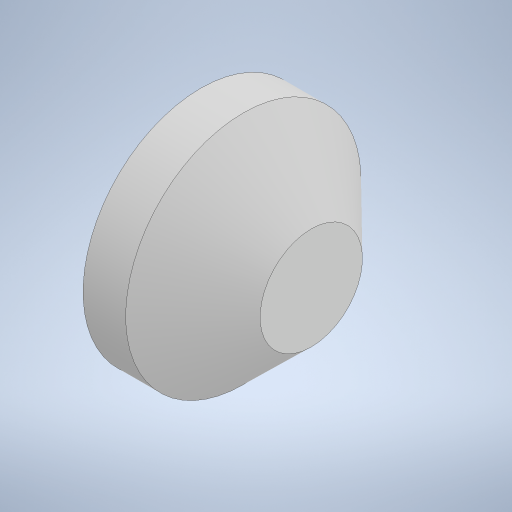
# Autodesk Inventor part: Part4
Saved by Autodesk Inventor 2023.2 (Build 272271030, 271C)
## iProperties
Created: 2024-03-05
Part Number: Part4
Material: Generic
Document SubType Name: Modeling
Designer: ryanv
Density: 1 g/cm^3
Appearance: Default
Author: ryanv
Autodesk Inventor part; units mm, degrees
ref_plane "YZ Plane" through (0, 0, 0) normal (1, 0, 0) x (0, 1, 0)
ref_plane "XZ Plane" through (0, 0, 0) normal (0, 1, 0) x (-1, 0, 0)
ref_plane "XY Plane" through (0, 0, 0) normal (0, 0, 1) x (1, 0, 0)
sketch "Sketch1" plane through (0, 0, 0) normal (0, 0, 1) x (1, 0, 0)
  line L0 (0, 0) -> (0, 12.4962)
  line L1 (0, 12.4962) -> (11.7356, 12.4962)
  line L2 (11.7356, 12.4962) -> (11.7356, 7.0631)
  line L3 (11.7356, 7.0631) -> (4.5276, 0)
  line L4 (4.5276, 0) -> (0, 0)
  constraints: 10 end point, 2 perpendicular, 1 parallel, 1 vertical
revolve "Revolution1" add sketch "Sketch1" angle 360 about axis through (0, 12.4962, 0) along (1, 0, 0)
body "Solid1"
